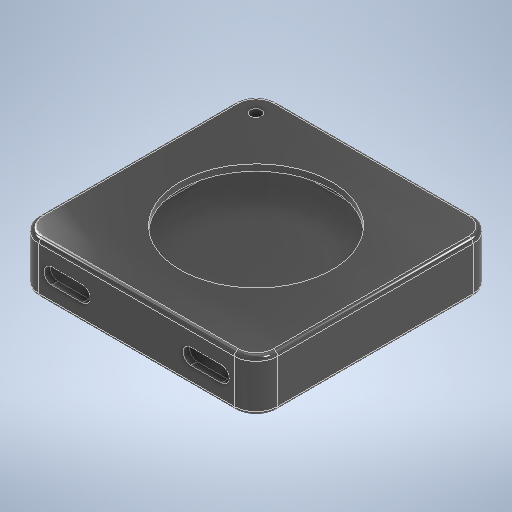
# Autodesk Inventor part: Box
Saved by Autodesk Inventor 2026 (Build 300175050, 175E)
## iProperties
Created: 2025-07-10
Part Number: Box
Material: Generic
Document SubType Name: Modeling
Designer: Jochen Alt
Density: 1 g/cm^3
Appearance: Default
Author: Jochen Alt
Autodesk Inventor part; units mm, degrees
ref_plane "YZ Plane" through (0, 0, 0) normal (1, 0, 0) x (0, 1, 0)
ref_plane "XZ Plane" through (0, 0, 0) normal (0, 1, 0) x (-1, 0, 0)
ref_plane "XY Plane" through (0, 0, 0) normal (0, 0, 1) x (1, 0, 0)
sketch "Sketch1" plane through (0, 0, 0) normal (0, 0, 1) x (1, 0, 0)
  line L0 (0, 38.5) -> (0, -38.5) construction
  line L1 (-38.5, 0) -> (38.5, 0) construction
  line L2 (-27.5, 27.5) -> (27.5, 27.5)
  line L3 (27.5, 27.5) -> (27.5, -27.5)
  line L4 (27.5, -27.5) -> (-27.5, -27.5)
  line L5 (-27.5, -27.5) -> (-27.5, 27.5)
  circle A0 centre (0, 0) radius 17.5
  dimension "d1" = 55
  dimension "d2" = 55
  dimension "d25" = 35
  constraints: 8 end point, 2 parallel, 1 centre point, 1 coincident, 1 horizontal, 1 perpendicular, 2 other
  measures "d1" distance between parallel lines of L3 L5
  measures "d2" distance between parallel lines of L4 L2
  measures "d25" diameter of A0
extrude "Extrusion1" add sketch "Sketch1" along normal blind 12 contours L2 L3 L4 L5 | A0
fillet "Fillet1" radius 5 4 edges at (-27.5, -27.5, 6) (27.5, -27.5, 6) (27.5, 27.5, 6) (-27.5, 27.5, 6)
fillet "Fillet2" radius 1 16 edges at (-26.0355, 26.0355, 12) (-27.5, 0, 12) (-26.0355, -26.0355, 12) (0, -27.5, 12) (26.0355, -26.0355, 12) (27.5, 0, 12) (26.0355, 26.0355, 12) (0, 27.5, 12) (-26.0355, 26.0355, 0) (-27.5, 0, 0) (-26.0355, -26.0355, 0) (0, -27.5, 0) (26.0355, -26.0355, 0) (27.5, 0, 0) (26.0355, 26.0355, 0) (0, 27.5, 0)
shell "Shell2" thickness 1.5 removed faces 0
sketch "USBPort" plane through (0, 0, 0) normal (0, 1, 0) x (-1, 0, 0)
  line L0 (19.5, 6) -> (12.5, 6) construction
  line L1 (19.5, 4.2) -> (12.5, 4.2)
  line L2 (12.5, 7.8) -> (19.5, 7.8)
  arc A0 (19.5, 4.2) -> (19.5, 7.8) centre (19.5, 6) ccw
  arc A1 (12.5, 7.8) -> (12.5, 4.2) centre (12.5, 6) ccw
  line L3 (-29.46, 0) -> (29.76, 0) construction
  line L4 (0, -1.56) -> (0, 9.36) construction
  circle A2 centre (-18, 6) radius 1
  line L5 (-19.5, 4.2) -> (-12.5, 4.2)
  line L6 (-12.5, 7.8) -> (-19.5, 7.8)
  arc A3 (-19.5, 7.8) -> (-19.5, 4.2) centre (-19.5, 6) ccw
  arc A4 (-12.5, 4.2) -> (-12.5, 7.8) centre (-12.5, 6) ccw
  point P0 (0, 0)
  point P1 (16, 6)
  dimension "d16" = 6
  dimension "d17" = 7
  dimension "d18" = 16
  dimension "d19" = 1.8
  dimension "d20" = 2
  dimension "d21" = 6
  dimension "d22" = 18
  constraints: 12 end point, 8 point on circle, 6 symmetric about line, 5 centre point, 4 tangent, 1 horizontal, 1 midpoint, 1 parallel, 2 other
  measures "d16" distance between parallel lines of L3 L0
  measures "d17" distance of L0.start L0.end
  measures "d18" distance from line of L4 point (16, 6)
  measures "d19" radius of A1
  measures "d20" diameter of A2
  measures "d21" distance from line of L3 A2.centre
  measures "d22" distance from line of L4 A2.centre
extrude "USB Port" cut sketch "USBPort" against normal up to next contours L1 A1 L2 A0 | A2 | A3 L6 A4 L5
extrude "Extrusion5" cut sketch "USBPort" along normal up to next contours A2
extrude "Extrusion6" cut sketch "Sketch1" against normal blind 5 from surface at 12 contours A0
sketch "Sketch3" plane through (0, 0, 0) normal (0, 0, 1) x (1, 0, 0)
  line L0 (0, 38.5) -> (0, -38.5) construction
  line L1 (-38.5, 0) -> (38.5, 0) construction
  circle A0 centre (-22.5, 22.5) radius 1.25
  line L2 (-27.5, 27.5) -> (27.5, 27.5) construction
  line L3 (-27.5, -27.5) -> (-27.5, 27.5) construction
  line L4 (27.5, -27.5) -> (-27.5, -27.5) construction
  line L5 (27.5, 27.5) -> (27.5, -27.5) construction
  point P0 (0, 0)
  dimension "d28" = 2.5
  dimension "d31" = 5
  dimension "d32" = 5
  constraints: 1 centre point
  measures "d28" diameter of A0
  measures "d31" distance from line of L2 A0.centre
  measures "d32" distance from line of A0.centre L3
extrude "Extrusion7" cut sketch "Sketch3" along normal blind 5 from surface at 10.5
equation "\"d2\" = d1"
equation "\"d21\" = d16"
equation "\"d32\" = d31"
body "Solid1"
